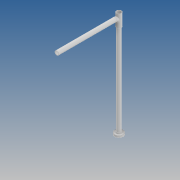
# Autodesk Inventor part: Slo
Saved by Autodesk Inventor 2020 (Build 240168000, 168)
## iProperties
Created: 2019-09-25
Part Number: Slo
Material: Generic
Document SubType Name: Modeling
Designer: a.komeijani
Density: 1 g/cm^3
Appearance: Default
Author: a.komeijani
Autodesk Inventor part; units mm, degrees
ref_plane "YZ Plane" through (0, 0, 0) normal (1, 0, 0) x (0, 1, 0)
ref_plane "XZ Plane" through (0, 0, 0) normal (0, 1, 0) x (-1, 0, 0)
ref_plane "XY Plane" through (0, 0, 0) normal (0, 0, 1) x (1, 0, 0)
sketch "Sketch1" plane through (0, 0, 0) normal (0, 1, 0) x (-1, 0, 0)
  circle A0 centre (0, 0) radius 100
  dimension "d0" = 200
  constraints: 1 centre point, 1 coincident
  measures "d0" diameter of A0
extrude "Extrusion1" add sketch "Sketch1" along normal blind 50
sketch "Sketch2" plane through (0, 0, 0) normal (0, -1, 0) x (1, 0, 0)
  circle A0 centre (0, 0) radius 90
  dimension "d3" = 180
  constraints: 1 centre point, 1 coincident
  measures "d3" diameter of A0
extrude "Extrusion2" cut sketch "Sketch2" against normal blind 30
sketch "Sketch3" plane through (0, 0, 0) normal (1, 0, 0) x (0, 1, 0)
  line L0 (0, 0) -> (10, 0)
  line L1 (10, 0) -> (10, -30)
  line L2 (10, -30) -> (0, -30)
  line L3 (0, -30) -> (0, 0)
  dimension "d6" = 10
  dimension "d7" = 30
  constraints: 8 end point, 2 parallel, 1 horizontal, 1 perpendicular
  measures "d6" distance of L1.end L2.end
  measures "d7" distance of L2.end L0.start
extrude "Extrusion3" cut sketch "Sketch3" against normal blind 400
pattern_circular "Circular Pattern1" count 12 over 360 about axis through (0, -10, 0) along (0, 1, 0) of "Extrusion3"
sketch "Sketch4" plane through (0, 50, 0) normal (0, 1, 0) x (1, 0, 0)
  circle A0 centre (0, 0) radius 60
  dimension "d13" = 120
  constraints: 1 centre point, 1 coincident
  measures "d13" diameter of A0
extrude "Extrusion4" add sketch "Sketch4" along normal blind 30
sketch "Sketch5" plane through (0, 80, 0) normal (0, 1, 0) x (1, 0, 0)
  circle A0 centre (0, 0) radius 50
  dimension "d16" = 100
  constraints: 1 centre point, 1 coincident
  measures "d16" diameter of A0
extrude "Extrusion5" cut sketch "Sketch5" against normal blind 20
sketch "Sketch6" plane through (0, 60, 0) normal (0, 1, 0) x (1, 0, 0)
  circle A0 centre (0, 0) radius 45
  dimension "d19" = 90
  constraints: 1 centre point, 1 coincident
  measures "d19" diameter of A0
extrude "Extrusion6" cut sketch "Sketch6" against normal blind 50
chamfer "Chamfer1" distance 20 angle 45 1 edges at (-45, 30, 0)
sketch "Sketch7" plane through (0, 60, 0) normal (0, 1, 0) x (1, 0, 0)
  circle A0 centre (0, 0) radius 50
  circle A1 centre (0, 0) radius 50 projected
  circle A2 centre (0, 0) radius 40
  dimension "d25" = 100
  dimension "d26" = 80
  constraints: 2 centre point, 2 coincident
  measures "d25" diameter of A0
  measures "d26" diameter of A2
extrude "Extrusion7" add sketch "Sketch7" along normal blind 2200
sketch "Sketch8" plane through (0, 2260, 0) normal (0, 1, 0) x (1, 0, 0)
  circle A0 centre (0, 0) radius 40 projected
  circle A1 centre (0, 0) radius 50
  circle A2 centre (0, 0) radius 40
  dimension "d29" = 100
  dimension "d30" = 80
  constraints: 2 centre point, 2 coincident
  measures "d29" diameter of A1
  measures "d30" diameter of A2
sketch "Sketch9" plane through (0, 0, 0) normal (1, 0, 0) x (0, 1, 0)
  line L0 (2260, -50) -> (2260, 50) projected
  line L1 (2260, 0) -> (2360, 0)
  line L2 (2460, 100) -> (2460, 1500)
  arc A0 (2360, 0) -> (2460, 100) centre (2360, 100) ccw
  point P0 (0, 0)
  point P1 (2460, 0)
  dimension "d34" = 200
  dimension "d35" = 1500
  dimension "d36" = 100
  constraints: 4 end point, 2 point on circle, 2 point on line, 2 tangent, 1 centre point, 1 horizontal, 1 midpoint, 1 vertical
  measures "d34" distance of L1.start point (2460, 0)
  measures "d35" distance of point (2460, 0) L2.end
  measures "d36" radius of A0
sweep "Sweep1" add profiles "Sketch8" path "Sketch9" path curves L1 A0 L2
ref_plane "Work Plane1" through (0, 2269.1625, 0) normal (0, 1, 0) x (1, 0, 0)
sketch "Sketch11" plane through (0, 2269.1625, 0) normal (0, 1, 0) x (1, 0, 0)
  circle A0 centre (0, 0) radius 40 projected
  circle A1 centre (0, 0) radius 50
  circle A2 centre (0, 0) radius 60 projected
  circle A3 centre (0, 0) radius 40
  dimension "d40" = 100
  dimension "d41" = 80
  constraints: 2 centre point, 2 coincident
  measures "d40" diameter of A1
  measures "d41" diameter of A3
extrude "Extrusion8" add sketch "Sketch11" along normal blind 300 contours A2
sketch "Sketch12" plane through (0, 2569.1625, 0) normal (0, 1, 0) x (1, 0, 0)
  arc A0 (-58.4847, 68.4072) -> (-77.9423, 45) centre (0, 0) ccw projected
  circle A1 centre (0, 0) radius 40
  dimension "d44" = 80
  constraints: 1 centre point, 1 coincident
  measures "d44" diameter of A1
extrude "Extrusion9" cut sketch "Sketch12" against normal blind 600
body "Solid1"
